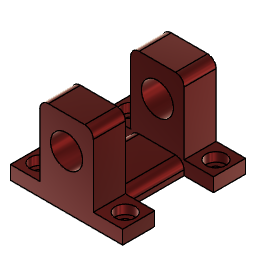
Soporte para Varilla (Autodesk Fusion 360 design; units mm, degrees)
Autodesk Fusion 360 part; units mm, degrees
sketch "Sketch1" plane through (0, 0, 0) normal (0, 0, 1) x (1, 0, 0)
  line L0 (9.8585, 2.8165) -> (-9.8585, 2.8165)
  line L1 (-9.8585, 2.8165) -> (-9.8585, -2.8165)
  line L2 (-9.8585, -2.8165) -> (9.8585, -2.8165)
  line L3 (9.8585, -2.8165) -> (9.8585, 2.8165)
  line L4 (9.8585, 2.8165) -> (-9.8585, -2.8165) construction
  line L5 (-9.8585, 2.8165) -> (9.8585, -2.8165) construction
  dimension "d1" = 19.717
  dimension "d2" = 5.633
  constraint horizontal L0
  constraint perpendicular L0 L1
  constraint parallel L0 L2
  constraint parallel L1 L3
  constraint coincident L4 origin
  constraint coincident L5 origin
  measures "d1" distance of L1.end L2.end
  measures "d2" distance of L0.end L1.end
extrude "Extrude1" add sketch "Sketch1" along normal blind 2.411 makes body 1
sketch "Sketch5" plane through (0, 0, 2.411) normal (0, 0, 1) x (-1, 0, 0)
  line L0 (-9.8585, 2.8165) -> (-9.8585, -2.8165)
  line L1 (-9.8585, -2.8165) -> (9.8585, -2.8165)
  line L2 (9.8585, -2.8165) -> (9.8585, 2.8165)
  line L3 (9.8585, 2.8165) -> (-9.8585, 2.8165)
  line L4 (0, -2.8165) -> (0, 2.8165) construction
  line L5 (9.8585, 0) -> (-9.8585, 0) construction
  point P0 (7.4845, 0)
  point P1 (-7.4845, 0)
  dimension "d16" = 2.374
  constraint midpoint L1 L4.start
  constraint midpoint L3 L4.end
  constraint midpoint L2 L5.start
  constraint midpoint L0 L5.end
  constraint coincident L5 P0
  constraint symmetric L4 P0 P1
  measures "d16" distance of L2 P0
sketch "Sketch2" plane through (0, 0, 2.411) normal (0, 0, 1) x (-1, 0, 0)
  line L0 (-9.8585, 2.8165) -> (-9.8585, -2.8165)
  line L1 (-9.8585, -2.8165) -> (9.8585, -2.8165)
  line L2 (9.8585, -2.8165) -> (9.8585, 2.8165)
  line L3 (9.8585, 2.8165) -> (-9.8585, 2.8165)
  line L4 (-4.6945, -2.8165) -> (4.6945, -2.8165)
  line L5 (4.6945, -2.8165) -> (4.6945, 2.8165)
  line L6 (4.6945, 2.8165) -> (-4.6945, 2.8165)
  line L7 (-4.6945, 2.8165) -> (-4.6945, -2.8165)
  line L8 (-4.6945, -2.8165) -> (4.6945, 2.8165) construction
  line L9 (4.6945, -2.8165) -> (-4.6945, 2.8165) construction
  dimension "d5" = 9.389
  constraint horizontal L4
  constraint perpendicular L4 L5
  constraint parallel L4 L6
  constraint parallel L5 L7
  constraint coincident L8 origin
  constraint coincident L9 origin
  measures "d5" distance of L5.end L6.end
sketch "Sketch3" plane through (0, -2.8165, 0) normal (0, -1, 0) x (1, 0, 0)
  line L0 (-9.8585, 0) -> (9.8585, 0)
  line L1 (9.8585, 0) -> (9.8585, 2.411)
  line L2 (9.8585, 2.411) -> (-9.8585, 2.411)
  line L3 (-9.8585, 2.411) -> (-9.8585, 0)
  line L4 (0, 2.411) -> (0, 0) construction
  line L5 (-4.6945, 2.411) -> (-4.6945, 0)
  line L6 (-4.6945, 0) -> (4.6945, 0)
  line L7 (4.6945, 0) -> (4.6945, 2.411)
  line L8 (4.6945, 2.411) -> (-4.6945, 0) construction
  line L9 (-4.6945, 2.411) -> (4.6945, 0) construction
  point P0 (0, 1.2055)
  dimension "d6" = 9.389
  constraint midpoint L2 L4.start
  constraint coincident L4.end origin
  constraint parallel L5 L7
  constraint coincident L8 P0
  constraint coincident L9 P0
  constraint midpoint L4 P0
  measures "d6" distance of L5.end L6.end
extrude "Extrude2" add sketch "Sketch2" along normal blind 12.581 contours L1 L3 L4 L5 L6 L7 bodies 1
sketch "Sketch4" plane through (0, -2.8165, 0) normal (0, -1, 0) x (1, 0, 0)
  line L0 (-9.8585, 0) -> (9.8585, 0)
  line L1 (9.8585, 0) -> (9.8585, 2.411)
  line L2 (9.8585, 2.411) -> (4.6945, 2.411)
  line L3 (4.6945, 2.411) -> (4.6945, 14.992)
  line L4 (4.6945, 14.992) -> (-4.6945, 14.992)
  line L5 (-4.6945, 14.992) -> (-4.6945, 2.411)
  line L6 (-4.6945, 2.411) -> (-9.8585, 2.411)
  line L7 (-9.8585, 2.411) -> (-9.8585, 0)
  line L8 (0, 14.992) -> (0, 2.5) construction
  point P0 (0, 9.358)
  dimension "d10" = 5.634
  constraint midpoint L4 L8.start
  constraint perpendicular L4 L8
  constraint coincident L8 P0
  measures "d10" distance of L4 P0
hole "Hole1" at (0, -2.8165, 9.358) direction (0, 1, 0) diameter 5.633 depth 5.633 tip angle 118 bodies 1
fillet "Fillet1" radius 1.5 2 edges at (4.6945, 0, 14.992) (-4.6945, 0, 14.992) on bodies 1
hole "Hole2" at (-7.4845, 0, 2.411) at (7.4845, 0, 2.411) direction (0, 0, -1) diameter 1.8 depth 3.5 tip angle 118 counterbore diameter 3.5 counterbore depth 1.6 bodies 1
copy_body "CopyPasteBodies1" bodies 1 makes body 2
move_body "Move1" bodies 2 to x (1, 0, 0) y (0, 1, 0) z (0, 0, 1) at (0, -15.961, 0)
extrude "Extrude3" add sketch "Sketch3" along normal up to surface (10.328 mm away) contours L0 L2 L5 L6 L7 bodies 1 2
fillet "Fillet2" radius 1.5 2 edges at (-4.6945, -7.9805, 2.411) (4.6945, -7.9805, 2.411) on bodies 1
